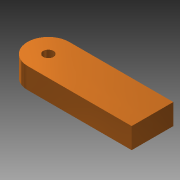
# Autodesk Inventor part: Base
Saved by Autodesk Inventor 2015 (Build 190159000, 159)
## iProperties
Created: 2016-11-08
Part Number: Base
Material: ゴールド
Document SubType Name: Modeling
Designer: MobileRoboMaster
Mass: 1756.21 g
Surface Area: 157.845 cm^2
Volume: 90.9956 cm^3
Density: 19.3 g/cm^3
Appearance: メタル 1600F 熱
Author: MobileRoboMaster
Autodesk Inventor part; units mm, degrees
ref_plane "YZ Plane" through (0, 0, 0) normal (1, 0, 0) x (0, 1, 0)
ref_plane "XZ Plane" through (0, 0, 0) normal (0, 1, 0) x (-1, 0, 0)
ref_plane "XY Plane" through (0, 0, 0) normal (0, 0, 1) x (1, 0, 0)
sketch "スケッチ1" plane through (0, 0, 0) normal (0, 0, 1) x (1, 0, 0)
  line L0 (0, 20) -> (100, 20)
  line L1 (100, 20) -> (100, -20)
  line L2 (100, -20) -> (0, -20)
  line L3 (0, -20) -> (0, 20)
  circle A0 centre (0, 0) radius 20
  dimension "d0" = 100
  dimension "d1" = 40
  dimension "d2" = 20
  dimension "d3" = 100
  constraints: 8 end point, 2 parallel, 1 coincident, 1 horizontal, 1 perpendicular, 1 vertical alignment, 2 other
  measures "d0" distance of L0.start L0.end
  measures "d1" distance of L2.end L0.start
  measures "d2" distance from line of point (0, 0) L2
  measures "d3" distance from line of point (0, 0) L1
extrude "押し出し1" add sketch "スケッチ1" along normal mid plane 20
sketch "スケッチ2" plane through (0, 0, 10) normal (0, 0, 1) x (1, 0, 0)
  circle A0 centre (0, 0) radius 5
  dimension "d6" = 10
  constraints: 1 centre point, 1 coincident
  measures "d6" diameter of A0
extrude "押し出し2" cut sketch "スケッチ2" against normal through all
equation "\"d2\" = 0.5 * d1"
equation "\"d3\" = d0"
equation "\"d7\" = d6"
